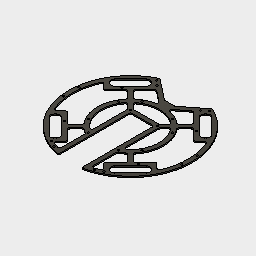
Middle Plate (Autodesk Fusion 360 design; units mm, degrees)
Autodesk Fusion 360 part; units mm, degrees
sketch "Sketch1" plane through (0, 0, 0) normal (0, 1, 0) x (1, 0, 0)
  circle A0 centre (-63.2861, 49.1439) radius 1.55
  circle A1 centre (63.2861, 49.1439) radius 1.55
  circle A2 centre (-63.2861, -49.1439) radius 1.55
  circle A3 centre (63.2861, -49.1439) radius 1.55
  arc A4 (45.2548, -72.1249) -> (45.2548, -80.6102) centre (49.4975, -76.3675) ccw
  circle A5 centre (25.9155, -45.8559) radius 1.55
  arc A6 (80.6102, -45.2548) -> (72.1249, -45.2548) centre (76.3675, -49.4975) ccw
  arc A7 (47.3762, -82.7315) -> (55.8614, -82.7315) centre (51.6188, -78.4889) ccw
  arc A8 (82.7315, -55.8614) -> (82.7315, -47.3762) centre (78.4889, -51.6188) ccw
  arc A9 (38.8918, -89.9524) -> (39.8226, -85.0774) centre (37.7012, -87.1987) ccw
  arc A10 (-33.234, -78.4889) -> (-33.234, -74.2462) centre (-35.3553, -76.3675) ccw
  arc A11 (-39.8226, -85.0774) -> (-38.8918, -89.9524) centre (-37.7012, -87.1987) ccw
  arc A12 (-58.3363, -49.1439) -> (-54.0937, -49.1439) centre (-56.215, -47.0226) ccw
  arc A13 (-49.1439, -54.0937) -> (-49.1439, -58.3363) centre (-47.0226, -56.215) ccw
  arc A14 (-35.1163, -43.8426) -> (-39.1131, -44.0628) centre (-36.9917, -46.1841) ccw
  circle A15 centre (-44.8286, -89.3777) radius 1.55
  arc A16 (54.0937, -49.1439) -> (58.3363, -49.1439) centre (56.215, -47.0226) ccw
  circle A17 centre (44.8286, -89.3777) radius 1.55
  arc A18 (-89.9524, 38.8918) -> (-89.9524, -38.8918) centre (0, 0) ccw
  arc A19 (-89.9524, -38.8918) -> (-85.0774, -39.8226) centre (-87.1987, -37.7012) ccw
  arc A20 (49.1439, 54.0937) -> (49.1439, 58.3363) centre (47.0226, 56.215) ccw
  line L0 (54.0937, 49.1439) -> (44.0628, 39.1131)
  line L1 (78.4889, 33.234) -> (85.0774, 39.8226)
  line L2 (-9.7255, 67.6367) -> (-43.2519, 93.8511)
  arc A21 (45.2548, 80.6102) -> (45.2548, 72.1249) centre (49.4975, 76.3675) ccw
  circle A22 centre (25.9155, 45.8559) radius 1.55
  circle A23 centre (45.8559, 25.9155) radius 1.55
  arc A24 (35.1163, 43.8426) -> (39.1131, 44.0628) centre (36.9917, 46.1841) ccw
  arc A25 (44.0628, 39.1131) -> (43.8426, 35.1163) centre (46.1841, 36.9917) ccw
  circle A26 centre (44.8298, 89.3777) radius 1.55
  arc A27 (35.1163, 43.8426) -> (12.5512, 54.7521) centre (0, 0) ccw
  arc A28 (33.4919, 73.9883) -> (29.5227, 74.2303) centre (31.3706, 71.867) ccw
  line L3 (-49.1439, 54.0937) -> (-39.1131, 44.0628)
  arc A29 (-43.8426, 35.1163) -> (-44.0628, 39.1131) centre (-46.1841, 36.9917) ccw
  arc A30 (-54.0937, 49.1439) -> (-58.3363, 49.1439) centre (-56.215, 47.0226) ccw
  arc A31 (-49.1439, 58.3363) -> (-49.1439, 54.0937) centre (-47.0226, 56.215) ccw
  arc A32 (-39.1131, 44.0628) -> (-35.1163, 43.8426) centre (-36.9917, 46.1841) ccw
  circle A33 centre (-45.8559, 25.9155) radius 1.55
  line L4 (-47.3762, 82.7315) -> (-45.2548, 80.6102)
  line L5 (-49.1439, 58.3363) -> (-33.4919, 73.9883)
  arc A34 (-43.2519, 93.8511) -> (-46.4263, 94.1785) centre (-45.0998, 91.4877) ccw
  circle A35 centre (-44.8298, 89.3777) radius 1.55
  arc A36 (-47.3762, 82.7315) -> (-55.8614, 82.7315) centre (-51.6188, 78.4889) ccw
  arc A37 (-45.2548, 72.1249) -> (-45.2548, 80.6102) centre (-49.4975, 76.3675) ccw
  line L6 (-45.2548, 72.1249) -> (-72.1249, 45.2548)
  line L7 (58.3363, 49.1439) -> (74.2462, 33.234)
  line L8 (55.8614, 82.7315) -> (69.2965, 69.2965)
  line L9 (82.7315, 47.3762) -> (80.6102, 45.2548)
  line L10 (69.2965, 69.2965) -> (82.7315, 55.8614)
  line L11 (72.1249, 45.2548) -> (45.2548, 72.1249)
  line L12 (29.5227, 74.2303) -> (11.3737, 60.0396)
  line L13 (49.1439, 58.3363) -> (33.4919, 73.9883)
  line L14 (43.2519, 93.8511) -> (9.7255, 67.6367)
  line L15 (-58.3363, -49.1439) -> (-74.2462, -33.234)
  line L16 (-49.1439, -58.3363) -> (-33.234, -74.2462)
  line L17 (-45.2548, -80.6102) -> (-47.3762, -82.7315)
  line L18 (-72.1249, -45.2548) -> (-45.2548, -72.1249)
  line L19 (-82.7315, -47.3762) -> (-80.6102, -45.2548)
  line L20 (-55.8614, -82.7315) -> (-69.2965, -69.2965)
  line L21 (-69.2965, -69.2965) -> (-82.7315, -55.8614)
  circle A38 centre (45.8559, -25.9155) radius 1.55
  arc A39 (89.9524, -38.8918) -> (89.9524, 38.8918) centre (0, 0) ccw
  arc A40 (78.4889, -33.234) -> (74.2462, -33.234) centre (76.3675, -35.3553) ccw
  arc A41 (85.0774, -39.8226) -> (89.9524, -38.8918) centre (87.1987, -37.7012) ccw
  arc A42 (43.8426, -35.1163) -> (43.8426, 35.1163) centre (0, 0) ccw
  arc A43 (43.8426, -35.1163) -> (44.0628, -39.1131) centre (46.1841, -36.9917) ccw
  circle A44 centre (100.6317, -13.2484) radius 1.55
  line L22 (85.0774, -39.8226) -> (78.4889, -33.234)
  line L23 (58.3363, -49.1439) -> (74.2462, -33.234)
  arc A45 (33.234, -74.2462) -> (33.234, -78.4889) centre (35.3553, -76.3675) ccw
  arc A46 (39.1131, -44.0628) -> (35.1163, -43.8426) centre (36.9917, -46.1841) ccw
  arc A47 (49.1439, -58.3363) -> (49.1439, -54.0937) centre (47.0226, -56.215) ccw
  line L24 (49.1439, 54.0937) -> (39.1131, 44.0628)
  line L25 (45.2548, 80.6102) -> (47.3762, 82.7315)
  arc A48 (55.8614, 82.7315) -> (47.3762, 82.7315) centre (51.6188, 78.4889) ccw
  arc A49 (82.7315, 47.3762) -> (82.7315, 55.8614) centre (78.4889, 51.6188) ccw
  arc A50 (72.1249, 45.2548) -> (80.6102, 45.2548) centre (76.3675, 49.4975) ccw
  arc A51 (89.9524, 38.8918) -> (85.0774, 39.8226) centre (87.1987, 37.7012) ccw
  arc A52 (-45.2548, -80.6102) -> (-45.2548, -72.1249) centre (-49.4975, -76.3675) ccw
  arc A53 (-82.7315, -47.3762) -> (-82.7315, -55.8614) centre (-78.4889, -51.6188) ccw
  arc A54 (-55.8614, -82.7315) -> (-47.3762, -82.7315) centre (-51.6188, -78.4889) ccw
  circle A55 centre (-25.9155, -45.8559) radius 1.55
  line L26 (-54.0937, -49.1439) -> (-44.0628, -39.1131)
  line L27 (-49.1439, -54.0937) -> (-39.1131, -44.0628)
  line L28 (-39.8226, -85.0774) -> (-33.234, -78.4889)
  circle A56 centre (-25.9155, 45.8559) radius 1.55
  arc A57 (-12.5512, 54.7521) -> (-35.1163, 43.8426) centre (0, 0) ccw
  arc A58 (-29.5227, 74.2303) -> (-33.4919, 73.9883) centre (-31.3706, 71.867) ccw
  arc A59 (-74.2462, -33.234) -> (-78.4889, -33.234) centre (-76.3675, -35.3553) ccw
  arc A60 (-43.8426, 35.1163) -> (-43.8426, -35.1163) centre (0, 0) ccw
  arc A61 (-44.0628, -39.1131) -> (-43.8426, -35.1163) centre (-46.1841, -36.9917) ccw
  circle A62 centre (-100.6317, -13.2484) radius 1.55
  line L29 (-78.4889, -33.234) -> (-85.0774, -39.8226)
  arc A63 (-72.1249, -45.2548) -> (-80.6102, -45.2548) centre (-76.3675, -49.4975) ccw
  line L30 (45.2548, -72.1249) -> (72.1249, -45.2548)
  line L31 (47.3762, -82.7315) -> (45.2548, -80.6102)
  line L32 (82.7315, -55.8614) -> (69.2965, -69.2965)
  line L33 (69.2965, -69.2965) -> (55.8614, -82.7315)
  line L34 (54.0937, -49.1439) -> (44.0628, -39.1131)
  line L35 (49.1439, -54.0937) -> (39.1131, -44.0628)
  line L36 (33.234, -78.4889) -> (39.8226, -85.0774)
  line L37 (49.1439, -58.3363) -> (33.234, -74.2462)
  line L38 (80.6102, -45.2548) -> (82.7315, -47.3762)
  arc A64 (-12.5512, 54.7521) -> (-11.3737, 60.0396) centre (-13.2216, 57.6763) ccw
  arc A65 (11.3737, 60.0396) -> (12.5512, 54.7521) centre (13.2216, 57.6763) ccw
  arc A66 (-9.7255, 67.6367) -> (-7.8776, 67) centre (-7.8776, 70) ccw
  arc A67 (7.8776, 67) -> (9.7255, 67.6367) centre (7.8776, 70) ccw
  line L39 (-29.5227, 74.2303) -> (-11.323, 60)
  line L40 (-11.323, 60) -> (-11.3737, 60.0396)
  line L41 (7.8776, 67) -> (-7.8776, 67)
  line L42 (-54.0937, 49.1439) -> (-44.0628, 39.1131)
  arc A68 (46.4263, 94.1785) -> (43.2519, 93.8511) centre (45.0998, 91.4877) ccw
  circle A69 centre (-45.8559, -25.9155) radius 1.55
  arc A70 (74.2462, 33.234) -> (78.4889, 33.234) centre (76.3675, 35.3553) ccw
  arc A71 (58.3363, 49.1439) -> (54.0937, 49.1439) centre (56.215, 47.0226) ccw
  arc A72 (-80.6102, 45.2548) -> (-72.1249, 45.2548) centre (-76.3675, 49.4975) ccw
  arc A73 (-82.7315, 55.8614) -> (-82.7315, 47.3762) centre (-78.4889, 51.6188) ccw
  arc A74 (-85.0774, 39.8226) -> (-89.9524, 38.8918) centre (-87.1987, 37.7012) ccw
  arc A75 (-78.4889, 33.234) -> (-74.2462, 33.234) centre (-76.3675, 35.3553) ccw
  line L43 (-85.0774, 39.8226) -> (-78.4889, 33.234)
  line L44 (-58.3363, 49.1439) -> (-74.2462, 33.234)
  line L45 (-80.6102, 45.2548) -> (-82.7315, 47.3762)
  line L46 (-82.7315, 55.8614) -> (-69.2965, 69.2965)
  line L47 (-69.2965, 69.2965) -> (-55.8614, 82.7315)
  line L48 (-20, -100.6231) -> (-20, 17)
  line L49 (-17, 20) -> (17, 20)
  line L50 (20, 17) -> (20, -100.6231)
  line L51 (34.7985, 29.8487) -> (27.8787, 22.9289)
  line L52 (29.8487, 34.7985) -> (22.9289, 27.8787)
  line L53 (-34.7985, 29.8487) -> (-27.8787, 22.9289)
  line L54 (-29.8487, 34.7985) -> (-22.9289, 27.8787)
  arc A76 (28.479, -48.4177) -> (35.1163, -43.8426) centre (0, 0) ccw
  arc A77 (-35.1163, -43.8426) -> (-28.479, -48.4177) centre (0, 0) ccw
  arc A78 (-38.8918, -89.9524) -> (-30.9474, -92.9853) centre (0, 0) ccw
  arc A79 (30.9474, -92.9853) -> (38.8918, -89.9524) centre (0, 0) ccw
  line L55 (-27, -90.1388) -> (-27, -51.0036)
  line L56 (-27, 20.8076) -> (-27, -35.0982)
  line L57 (27, -51.0036) -> (27, -90.1388)
  line L58 (27, 20.8076) -> (27, -35.0982)
  line L59 (20.8076, 27) -> (-20.8076, 27)
  arc A80 (-31.9492, -37.3787) -> (-27, -35.0982) centre (-30, -35.0982) ccw
  arc A81 (-27, -51.0036) -> (-28.479, -48.4177) centre (-30, -51.0036) ccw
  arc A82 (-30.9474, -92.9853) -> (-27, -90.1388) centre (-30, -90.1388) ccw
  arc A83 (28.479, -48.4177) -> (27, -51.0036) centre (30, -51.0036) ccw
  arc A84 (27, -35.0982) -> (31.9492, -37.3787) centre (30, -35.0982) ccw
  arc A85 (-27, 20.8076) -> (-27.8787, 22.9289) centre (-30, 20.8076) ccw
  arc A86 (-17, 20) -> (-20, 17) centre (-17, 17) ccw
  arc A87 (20, 17) -> (17, 20) centre (17, 17) ccw
  arc A88 (27.8787, 22.9289) -> (27, 20.8076) centre (30, 20.8076) ccw
  arc A89 (-22.9289, 27.8787) -> (-20.8076, 27) centre (-20.8076, 30) ccw
  arc A90 (20.8076, 27) -> (22.9289, 27.8787) centre (20.8076, 30) ccw
  arc A91 (-39.3186, 29.529) -> (-31.9492, -37.3787) centre (0, 0) ccw
  arc A92 (31.9492, -37.3787) -> (39.3186, 29.529) centre (0, 0) ccw
  arc A93 (29.529, 39.3186) -> (-29.529, 39.3186) centre (0, 0) ccw
  arc A94 (-34.7985, 29.8487) -> (-39.3186, 29.529) centre (-36.9198, 27.7274) ccw
  arc A95 (-29.529, 39.3186) -> (-29.8487, 34.7985) centre (-27.7274, 36.9198) ccw
  arc A96 (29.8487, 34.7985) -> (29.529, 39.3186) centre (27.7274, 36.9198) ccw
  arc A97 (39.3186, 29.529) -> (34.7985, 29.8487) centre (36.9198, 27.7274) ccw
  arc A98 (-22.4272, -102.5769) -> (-20, -100.6231) centre (-22, -100.6231) ccw
  arc A99 (20, -100.6231) -> (22.4272, -102.5769) centre (22, -100.6231) ccw
  arc A100 (27, -90.1388) -> (30.9474, -92.9853) centre (30, -90.1388) ccw
  circle A101 centre (-23, 23.5) radius 1.55
  circle A102 centre (23, 23.5) radius 1.55
  arc A103 (-46.4263, 94.1785) -> (-22.4272, -102.5769) centre (0, 0) ccw
  arc A104 (22.4272, -102.5769) -> (46.4263, 94.1785) centre (0, 0) ccw
  circle A105 centre (37, 82.5) radius 1.5
  circle A106 centre (-37, 82.5) radius 1.5
  circle A107 centre (-100.6317, 13.2484) radius 1.5
  circle A108 centre (100.6317, 13.2484) radius 1.5
  circle A109 centre (34.715, -95.3788) radius 1.5
  circle A110 centre (-34.715, -95.3788) radius 1.5
  point P0 (86.9741, 51.6188)
  point P1 (76.3675, 41.0122)
  point P2 (41.0122, 76.3675)
  point P3 (51.6188, 86.9741)
  point P4 (-86.9741, 51.6188)
  point P5 (-41.0122, 76.3675)
  point P6 (-51.6188, 86.9741)
  point P7 (-76.3675, 41.0122)
  point P8 (-51.6188, -86.9741)
  point P9 (-76.3675, -41.0122)
  point P10 (-86.9741, -51.6188)
  point P11 (-41.0122, -76.3675)
  point P12 (86.9741, -51.6188)
  point P13 (-31.1127, -76.3675)
  point P14 (41.0122, -76.3675)
  point P15 (51.6188, -86.9741)
  point P16 (76.3675, -41.0122)
  point P17 (20, -105)
  point P18 (-20, -105)
  dimension "d254" = 3
  dimension "d255" = 3
  dimension "d256" = 3
  dimension "d257" = 3
  dimension "d266" = 3
  dimension "d269" = 3
  measures "d254" diameter of A105
  measures "d255" diameter of A106
  measures "d256" diameter of A108
  measures "d257" diameter of A107
  measures "d266" diameter of A109
  measures "d269" diameter of A110
extrude "Extrude1" add sketch "Sketch1" along normal blind 2
